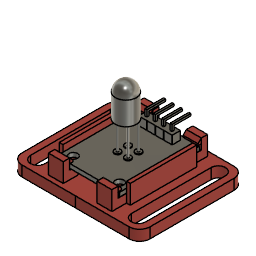
LED Holder (Autodesk Fusion 360 design; units mm, degrees)
Autodesk Fusion 360 part; units mm, degrees
note: some values were not read from the file. Chosen so that the rebuilt part matches the saved one: which bodies a step acts on; which face or edge a step refers to. Set by a fixed rule: which sketch regions a step uses.
sketch "Sketch1" plane through (0, 0, 0) normal (0, 0, 1) x (1, 0, 0)
  line L0 (0, 0) -> (15, 0)
  line L1 (15, 0) -> (15, 19)
  line L2 (15, 19) -> (0, 19)
  line L3 (0, 19) -> (0, 0)
  line L4 (0, 0) -> (2, 0) construction
  line L5 (2, 0) -> (2, 2) construction
  line L6 (2, 2) -> (0, 2) construction
  line L7 (0, 2) -> (0, 0) construction
  circle A0 centre (2, 2) radius 1
  circle A1 centre (13, 2) radius 1
  dimension "d1" = 15
  dimension "d2" = 19
  constraint horizontal L0
  constraint vertical L1
  constraint horizontal L2
  constraint vertical L3
  constraint coincident L0.start L3.end
  constraint horizontal L4
  constraint vertical L5
  constraint horizontal L6
  constraint vertical L7
  constraint coincident L5.end L6.start
  measures "d1" distance of L0.start L0.end
  measures "d2" distance of L0.start L2.end
extrude "Extrude1" add sketch "Sketch1" along normal blind 1 makes body 1
sketch "Sketch2" plane through (0, 0, 1) normal (0, 0, 1) x (-1, 0, 0)
  circle A0 centre (-13, -2) radius 1
  circle A1 centre (-2, -2) radius 1
  line L0 (0, -19) -> (0, 0)
  line L1 (0, 0) -> (-15, 0)
  line L2 (-15, 0) -> (-15, -19)
  line L3 (-15, -19) -> (0, -19)
  line L4 (-7.5, -19) -> (-7.5, -18) construction
  line L5 (-7.5, -18) -> (-7.5, -17) construction
  line L6 (-11.5, -18) -> (-3.5, -18)
  line L7 (-3.5, -18) -> (-3.5, -16)
  line L8 (-3.5, -16) -> (-11.5, -16)
  line L9 (-11.5, -16) -> (-11.5, -18)
  line L10 (-11.5, -18) -> (-3.5, -16) construction
  line L11 (-3.5, -18) -> (-11.5, -16) construction
  circle A2 centre (-3.5, -18) radius 0.05
  circle A3 centre (-5.5, -18) radius 0.05
  circle A4 centre (-7.5, -18) radius 0.05
  circle A5 centre (-9.5, -18) radius 0.05
  circle A6 centre (-11.5, -18) radius 0.05
  circle A7 centre (-3.5, -16) radius 0.05
  circle A8 centre (-5.5, -16) radius 0.05
  circle A9 centre (-7.5, -16) radius 0.05
  circle A10 centre (-9.5, -16) radius 0.05
  circle A11 centre (-11.5, -16) radius 0.05
  point P0 (-7.5, -17)
  dimension "d5" = 8
  dimension "d6" = 2
  dimension "d7" = 0.1
  dimension "d10" = -2
  dimension "d11" = 2
  constraint midpoint L3 L4.start
  constraint perpendicular L3 L4
  constraint parallel L4 L5
  constraint horizontal L6
  constraint perpendicular L6 L7
  constraint parallel L6 L8
  constraint parallel L7 L9
  constraint coincident L10 P0
  constraint coincident L11 P0
  constraint coincident P0 L5.end
  constraint coincident L6.end L7.start
  measures "d5" distance of L7.end L8.end
  measures "d6" distance of L6.end L7.end
  measures "d7" diameter of A2
extrude "Extrude2" add sketch "Sketch2" along normal blind 2 contours L6 L7 L8 L9 A2 A3 A4 A5 A6 A7 A8 A9 A10 A11 bodies 1
sketch "Sketch3" plane through (0, 0, 1) normal (0, 0, 1) x (-1, 0, 0)
  arc A0 (-7.55, -16) -> (-7.45, -16) centre (-7.5, -16) ccw
  line L0 (-7.45, -16) -> (-5.55, -16)
  arc A1 (-5.55, -16) -> (-5.45, -16) centre (-5.5, -16) ccw
  line L1 (-5.45, -16) -> (-3.55, -16)
  arc A2 (-3.55, -16) -> (-3.5, -16.05) centre (-3.5, -16) ccw
  line L2 (-3.5, -16.05) -> (-3.5, -17.95)
  arc A3 (-3.5, -17.95) -> (-3.55, -18) centre (-3.5, -18) ccw
  line L3 (-3.55, -18) -> (-5.45, -18)
  arc A4 (-5.45, -18) -> (-5.55, -18) centre (-5.5, -18) ccw
  line L4 (-5.55, -18) -> (-7.45, -18)
  arc A5 (-7.45, -18) -> (-7.55, -18) centre (-7.5, -18) ccw
  line L5 (-7.55, -18) -> (-9.45, -18)
  arc A6 (-9.45, -18) -> (-9.55, -18) centre (-9.5, -18) ccw
  line L6 (-9.55, -18) -> (-11.45, -18)
  arc A7 (-11.45, -18) -> (-11.5, -17.95) centre (-11.5, -18) ccw
  line L7 (-11.5, -17.95) -> (-11.5, -16.05)
  arc A8 (-11.5, -16.05) -> (-11.45, -16) centre (-11.5, -16) ccw
  line L8 (-11.45, -16) -> (-9.55, -16)
  arc A9 (-9.55, -16) -> (-9.45, -16) centre (-9.5, -16) ccw
  line L9 (-9.45, -16) -> (-7.55, -16)
  circle A10 centre (-13, -2) radius 1
  circle A11 centre (-2, -2) radius 1
  line L10 (0, -19) -> (0, 0)
  line L11 (0, 0) -> (-15, 0)
  line L12 (-15, 0) -> (-15, -19)
  line L13 (-15, -19) -> (0, -19)
  line L14 (-7.5, -19) -> (-7.5, -9) construction
  circle A12 centre (-7.5, -9) radius 2.5
  dimension "d14" = 10
  dimension "d15" = 5
  constraint midpoint L13 L14.start
  constraint perpendicular L13 L14
  constraint coincident L14.end A12.centre
  measures "d14" distance of L14.start L14.end
  measures "d15" diameter of A12
extrude "Extrude3" add sketch "Sketch3" along normal blind 15 contours A12 bodies 1
extrude "Extrude4" cut sketch "Sketch3" along normal blind 7 contours A12 bodies 1 makes body 2 at (5.8333, 13.622, 0)
fillet "Fillet1" radius 2.5 1 edges at (9.8308, 9.904, 16) on bodies 1
sketch "Sketch4" plane through (0, 0, 1) normal (0, 0, 1) x (-1, 0, 0)
  circle A0 centre (-6.5, -10.5) radius 0.75
  circle A1 centre (-6.5, -8) radius 0.75
  circle A2 centre (-9, -10.5) radius 0.75
  circle A3 centre (-9, -8) radius 0.75
  circle A4 centre (-6.5, -10.5) radius 0.25
  circle A5 centre (-6.5, -8) radius 0.25
  circle A6 centre (-9, -8) radius 0.25
  circle A7 centre (-9, -10.5) radius 0.25
  dimension "d22" = 1.5
  dimension "d23" = 1.5
  dimension "d24" = 1.5
  dimension "d25" = 1.5
  dimension "d26" = 0.5
  dimension "d27" = 0.5
  dimension "d28" = 0.5
  dimension "d29" = 0.5
  constraint concentric A0 A4
  constraint concentric A1 A5
  constraint concentric A3 A6
  constraint concentric A2 A7
  measures "d22" diameter of A0
  measures "d23" diameter of A1
  measures "d24" diameter of A2
  measures "d25" diameter of A3
  measures "d26" diameter of A4
  measures "d27" diameter of A5
  measures "d28" diameter of A6
  measures "d29" diameter of A7
extrude "Extrude5" add sketch "Sketch4" along normal blind 7 contours A4 | A5 | A6 | A7 bodies 1 2
extrude "Extrude7" add sketch "Sketch4" against normal blind 2 contours A4 | A5 | A6 | A7 bodies 1
extrude "Extrude8" add sketch "Sketch4" along normal blind 0.2 bodies 1
sketch "Sketch5" plane through (0, 0, 3) normal (0, 0, 1) x (-1, 0, 0)
  line L0 (-7.55, -16) -> (-9.45, -16)
  arc A0 (-9.55, -16) -> (-9.45, -16) centre (-9.5, -16) ccw
  line L1 (-9.55, -16) -> (-11.45, -16)
  arc A1 (-11.5, -16.05) -> (-11.45, -16) centre (-11.5, -16) ccw
  line L2 (-11.5, -16.05) -> (-11.5, -17.95)
  arc A2 (-11.45, -18) -> (-11.5, -17.95) centre (-11.5, -18) ccw
  line L3 (-11.45, -18) -> (-9.55, -18)
  arc A3 (-9.45, -18) -> (-9.55, -18) centre (-9.5, -18) ccw
  line L4 (-9.45, -18) -> (-7.55, -18)
  arc A4 (-7.45, -18) -> (-7.55, -18) centre (-7.5, -18) ccw
  line L5 (-7.45, -18) -> (-5.55, -18)
  arc A5 (-5.45, -18) -> (-5.55, -18) centre (-5.5, -18) ccw
  line L6 (-5.45, -18) -> (-3.55, -18)
  arc A6 (-3.5, -17.95) -> (-3.55, -18) centre (-3.5, -18) ccw
  line L7 (-3.5, -17.95) -> (-3.5, -16.05)
  arc A7 (-3.55, -16) -> (-3.5, -16.05) centre (-3.5, -16) ccw
  line L8 (-3.55, -16) -> (-5.45, -16)
  arc A8 (-5.55, -16) -> (-5.45, -16) centre (-5.5, -16) ccw
  line L9 (-5.55, -16) -> (-7.45, -16)
  arc A9 (-7.55, -16) -> (-7.45, -16) centre (-7.5, -16) ccw
  line L10 (-10.25, -16.75) -> (-10.75, -16.75)
  line L11 (-10.75, -16.75) -> (-10.75, -17.25)
  line L12 (-10.75, -17.25) -> (-10.25, -17.25)
  line L13 (-10.25, -17.25) -> (-10.25, -16.75)
  line L14 (-10.25, -16.75) -> (-10.75, -17.25) construction
  line L15 (-10.75, -16.75) -> (-10.25, -17.25) construction
  line L16 (-8.25, -17.25) -> (-8.25, -16.75)
  line L17 (-8.25, -16.75) -> (-8.75, -16.75)
  line L18 (-8.75, -16.75) -> (-8.75, -17.25)
  line L19 (-8.75, -17.25) -> (-8.25, -17.25)
  line L20 (-6.25, -17.25) -> (-6.25, -16.75)
  line L21 (-6.25, -16.75) -> (-6.75, -16.75)
  line L22 (-6.75, -16.75) -> (-6.75, -17.25)
  line L23 (-6.75, -17.25) -> (-6.25, -17.25)
  line L24 (-4.25, -17.25) -> (-4.25, -16.75)
  line L25 (-4.25, -16.75) -> (-4.75, -16.75)
  line L26 (-4.75, -16.75) -> (-4.75, -17.25)
  line L27 (-4.75, -17.25) -> (-4.25, -17.25)
  point P0 (-10.5, -17)
  dimension "d38" = 0.5
  dimension "d39" = 0.5
  dimension "d42" = 2
  dimension "d43" = 0
  constraint horizontal L10
  constraint perpendicular L10 L11
  constraint parallel L10 L12
  constraint parallel L11 L13
  constraint coincident L14 P0
  constraint coincident L15 P0
  measures "d38" distance of L11.end L12.end
  measures "d39" distance of L10.end L11.end
extrude "Extrude9" add sketch "Sketch5" along normal blind 1.5 contours L10 L11 L12 L13 | L16 L17 L18 L19 | L20 L21 L22 L23 | L24 L25 L26 L27 bodies 1
sketch "Sketch6" plane through (0, 17.25, 0) normal (0, 1, 0) x (-1, 0, 0)
  line L0 (-10.75, 3) -> (-10.25, 3)
  line L1 (-10.25, 3) -> (-10.25, 4.5)
  line L2 (-10.25, 4.5) -> (-10.75, 4.5)
  line L3 (-10.75, 4.5) -> (-10.75, 3)
  line L4 (-10.75, 4.5) -> (-10.25, 4.5)
  line L5 (-10.25, 4.5) -> (-10.25, 4)
  line L6 (-10.25, 4) -> (-10.75, 4)
  line L7 (-10.75, 4) -> (-10.75, 4.5)
  dimension "d46" = 0.5
  constraint horizontal L4
  constraint vertical L5
  constraint horizontal L6
  constraint vertical L7
  constraint coincident L2.end L3.start
  measures "d46" distance of L2.end L6.end
extrude "Extrude10" add sketch "Sketch6" along normal blind 4 contours L1 L2 L3 L4 L5 L6 L7 bodies 1
pattern_linear "R-Pattern1" count 4 spacing 2 along (-1, 0, 0) of "Extrude10"
sketch "Sketch7" plane through (0, 0, 0) normal (0, 0, -1) x (1, 0, 0)
  circle A0 centre (9, -10.5) radius 0.25
  circle A1 centre (9, -8) radius 0.25
  circle A2 centre (6.5, -10.5) radius 0.25
  circle A3 centre (6.5, -8) radius 0.25
  circle A4 centre (13, -2) radius 1
  circle A5 centre (2, -2) radius 1
  line L0 (0, 0) -> (0, -19)
  line L1 (0, -19) -> (15, -19)
  line L2 (15, -19) -> (15, 0)
  line L3 (15, 0) -> (0, 0)
  line L4 (7.5, 0) -> (-5.25, 0) construction
  line L5 (-5.25, 0) -> (7.5, 0)
  line L6 (7.5, -25) -> (-5.25, -25)
  line L7 (-7.75, -22.5) -> (-7.75, -2.5)
  line L8 (-7.75, -12.5) -> (-4.5, -12.5) construction
  line L9 (-2.8, -22) -> (-2.8, -3)
  arc A6 (-2.8, -3) -> (-6.2, -3) centre (-4.5, -3) ccw
  line L10 (-6.2, -3) -> (-6.2, -22)
  arc A7 (-6.2, -22) -> (-2.8, -22) centre (-4.5, -22) ccw
  line L11 (-4.5, -22) -> (-4.5, -3) construction
  line L12 (7.5, -25) -> (7.5, 0) construction
  arc A8 (-5.25, 0) -> (-7.75, -2.5) centre (-5.25, -2.5) ccw
  line L13 (0, 0) -> (7.5, 0) construction
  arc A9 (-7.75, -22.5) -> (-5.25, -25) centre (-5.25, -22.5) ccw
  line L14 (20.25, 0) -> (7.5, 0)
  arc A10 (22.75, -2.5) -> (20.25, 0) centre (20.25, -2.5) ccw
  line L15 (22.75, -22.5) -> (22.75, -2.5)
  arc A11 (20.25, -25) -> (22.75, -22.5) centre (20.25, -22.5) ccw
  line L16 (7.5, -25) -> (20.25, -25)
  arc A12 (17.8, -22) -> (21.2, -22) centre (19.5, -22) ccw
  line L17 (17.8, -22) -> (17.8, -3)
  line L18 (21.2, -3) -> (21.2, -22)
  arc A13 (21.2, -3) -> (17.8, -3) centre (19.5, -3) ccw
  line L19 (19.5, -22) -> (-4.5, -22) construction
  point P0 (-4.5, -12.5)
  dimension "d53" = 3.25
  dimension "d54" = 3.4
  dimension "d55" = 2.5
  dimension "d56" = 2.5
  dimension "d59" = 25
  dimension "d60" = 19
  dimension "d68" = 30.5
  dimension "d69" = 24
  constraint midpoint L3 L4.start
  constraint parallel L3 L4
  constraint perpendicular L2 L13
  constraint horizontal L5
  constraint horizontal L6
  constraint vertical L7
  constraint perpendicular L0 L8
  constraint tangent L9 A6
  constraint tangent A6 L10
  constraint parallel L9 L10
  constraint tangent L10 A7
  constraint tangent L9 A7
  constraint perpendicular L8 L11
  constraint coincident P0 L8.end
  constraint midpoint L11 P0
  constraint coincident L7 L8.start
  constraint tangent L5 A8
  constraint tangent L7 A8
  constraint coincident L0 L3.end
  constraint tangent L6 A9
  constraint tangent L7 A9
  constraint symmetric L4.start L12 L5.end
  constraint symmetric L9.start L12 A12.start
  constraint symmetric L9.end L12 L17.end
  constraint symmetric A6.end L12 L18.start
  constraint symmetric L10.end L12 A12.end
  constraint symmetric A6 L12 A13
  constraint symmetric A7 L12 A12
  constraint symmetric L6.start L12 L16.start
  constraint symmetric L12 L4.end L14.start
  constraint symmetric L12 L7.end A10.start
  constraint symmetric L12 A8 A10
  constraint symmetric L12 L6.end A11.start
  constraint symmetric L12 L7.start L15.start
  constraint symmetric L12 A9 A11
  constraint coincident A12.centre L19.start
  constraint coincident A7.centre L11.start
  measures "d53" distance of L8.start P0
  measures "d54" diameter of A6
  measures "d55" radius of A8
  measures "d56" radius of A9
  measures "d59" distance of L5 L6
  measures "d60" distance of A7.centre A6.centre
  measures "d68" distance of L7 L15
  measures "d69" distance of A12.centre A7.centre
extrude "Extrude11" add sketch "Sketch7" along normal blind 2.5 separate body contours A0 | A1 | A2 | A3 | A4 | A5 | L0 L1 L2 L3 L5 L14 | L0 L1 L2 L5 L6 L7 A8 A9 L14 A10 L15 A11 L16 makes body 3
move_body "Move1" bodies 1 to x (1, 0, 0) y (0, 1, 0) z (0, 0, 1) at (0, 3, 2)
sketch "Sketch8" plane through (0, 0, 0) normal (0, 0, 1) x (-1, 0, 0)
  arc A0 (2.8, -22) -> (6.2, -22) centre (4.5, -22) ccw
  line L0 (2.8, -22) -> (2.8, -3)
  arc A1 (6.2, -3) -> (2.8, -3) centre (4.5, -3) ccw
  line L1 (6.2, -3) -> (6.2, -22)
  arc A2 (-21.2, -22) -> (-17.8, -22) centre (-19.5, -22) ccw
  line L2 (-21.2, -22) -> (-21.2, -3)
  arc A3 (-17.8, -3) -> (-21.2, -3) centre (-19.5, -3) ccw
  line L3 (-17.8, -3) -> (-17.8, -22)
  arc A4 (5.25, -25) -> (7.75, -22.5) centre (5.25, -22.5) ccw
  line L4 (7.75, -22.5) -> (7.75, -2.5)
  arc A5 (7.75, -2.5) -> (5.25, 0) centre (5.25, -2.5) ccw
  line L5 (5.25, 0) -> (-7.5, 0)
  line L6 (-7.5, 0) -> (-20.25, 0)
  arc A6 (-20.25, 0) -> (-22.75, -2.5) centre (-20.25, -2.5) ccw
  line L7 (-22.75, -2.5) -> (-22.75, -22.5)
  arc A7 (-22.75, -22.5) -> (-20.25, -25) centre (-20.25, -22.5) ccw
  line L8 (-20.25, -25) -> (-7.5, -25)
  line L9 (-7.5, -25) -> (5.25, -25)
  line L10 (0.05, -20.4) -> (-3.5, -20.4)
  line L11 (-3.5, -20.4) -> (-3.5, -23.9)
  line L12 (-3.5, -23.9) -> (0.05, -23.9)
  line L13 (0.05, -23.9) -> (0.05, -20.4)
  line L14 (0.05, -23.9) -> (-3.5, -23.9)
  line L15 (-3.5, -23.9) -> (-3.5, -22.4)
  line L16 (-3.5, -22.4) -> (0.05, -22.4)
  line L17 (0.05, -22.4) -> (0.05, -23.9)
  line L18 (-7.5, -25) -> (-7.5, 0) construction
  line L19 (7.75, -12.5) -> (-22.75, -12.5) construction
  line L20 (-15.05, -20.4) -> (-11.5, -20.4)
  line L21 (-11.5, -20.4) -> (-11.5, -23.9)
  line L22 (-15.05, -23.9) -> (-15.05, -20.4)
  line L23 (-11.5, -23.9) -> (-15.05, -23.9)
  line L24 (-15.05, -23.9) -> (-11.5, -23.9)
  line L25 (-11.5, -23.9) -> (-11.5, -22.4)
  line L26 (-15.05, -22.4) -> (-15.05, -23.9)
  line L27 (-11.5, -22.4) -> (-15.05, -22.4)
  line L28 (0.05, -4.6) -> (-3.5, -4.6)
  line L29 (-3.5, -4.6) -> (-3.5, -1.1)
  line L30 (0.05, -1.1) -> (0.05, -4.6)
  line L31 (-3.5, -1.1) -> (0.05, -1.1)
  line L32 (0.05, -1.1) -> (-3.5, -1.1)
  line L33 (-3.5, -1.1) -> (-3.5, -2.6)
  line L34 (0.05, -2.6) -> (0.05, -1.1)
  line L35 (-3.5, -2.6) -> (0.05, -2.6)
  line L36 (-11.5, -1.1) -> (-11.5, -2.6)
  line L37 (-11.5, -2.6) -> (-15.05, -2.6)
  line L38 (-15.05, -2.6) -> (-15.05, -1.1)
  line L39 (-15.05, -1.1) -> (-11.5, -1.1)
  line L40 (-15.05, -1.1) -> (-15.05, -4.6)
  line L41 (-11.5, -4.6) -> (-11.5, -1.1)
  line L42 (-11.5, -1.1) -> (-15.05, -1.1)
  line L43 (-15.05, -4.6) -> (-11.5, -4.6)
  line L44 (0.05, -20.4) -> (0.95, -20.4)
  line L45 (0.95, -20.4) -> (0.95, -4.6)
  line L46 (0.95, -4.6) -> (0.05, -4.6)
  line L47 (0.05, -4.6) -> (0.05, -20.4)
  line L48 (0.05, -20.4) -> (0.95, -4.6) construction
  line L49 (0.95, -20.4) -> (0.05, -4.6) construction
  line L50 (-15.05, -20.4) -> (-15.95, -20.4)
  line L51 (-15.95, -20.4) -> (-15.95, -4.6)
  line L52 (-15.95, -4.6) -> (-15.05, -4.6)
  line L53 (-15.05, -4.6) -> (-15.05, -20.4)
  point P0 (0.5, -12.5)
  dimension "d70" = 0.9
  constraint horizontal L10
  constraint vertical L11
  constraint horizontal L12
  constraint vertical L13
  constraint horizontal L14
  constraint vertical L15
  constraint horizontal L16
  constraint vertical L17
  constraint coincident L8.end L9.start
  constraint coincident L5.end L6.start
  constraint midpoint L4 L19.start
  constraint midpoint L7 L19.end
  constraint symmetric L10.start L18 L20.start
  constraint symmetric L10.end L18 L20.end
  constraint symmetric L11.end L18 L21.end
  constraint symmetric L12.end L18 L22.start
  constraint symmetric L15.end L18 L25.end
  constraint symmetric L16.end L18 L26.start
  constraint symmetric L10.start L19 L28.start
  constraint symmetric L10.end L19 L28.end
  constraint symmetric L11.end L19 L29.end
  constraint symmetric L12.end L19 L30.start
  constraint symmetric L15.end L19 L33.end
  constraint symmetric L16.end L19 L34.start
  constraint symmetric L19 L20.start L40.end
  constraint symmetric L19 L20.end L41.start
  constraint symmetric L19 L21.end L36.start
  constraint symmetric L19 L22.start L38.end
  constraint symmetric L19 L25.end L36.end
  constraint symmetric L19 L26.start L37.end
  constraint horizontal L44
  constraint perpendicular L44 L45
  constraint parallel L44 L46
  constraint parallel L45 L47
  constraint coincident L48 P0
  constraint coincident L49 P0
  constraint coincident L19 P0
  constraint symmetric L18 L44.end L50.end
  constraint symmetric L18 L45.end L51.end
  constraint symmetric L18 L28.start L40.end
  measures "d70" distance of L45 L47
extrude "Extrude12" add sketch "Sketch8" along normal blind 2 contours L10 L11 L13 L16 | L28 L29 L30 L35 | L20 L21 L22 L27 | L37 L40 L41 L43 bodies 3
extrude "Extrude13" add sketch "Sketch8" along normal blind 4.5 contours L44 L45 L46 L47 | L11 L12 L13 L14 L15 L16 L17 | L29 L30 L31 L32 L33 L34 L35 | L50 L51 L52 L53 | L21 L22 L23 L24 L25 L26 L27 | L36 L37 L38 L39 L40 L41 L42 bodies 3
sketch "Sketch9" plane through (0, 0, 4.5) normal (0, 0, 1) x (-1, 0, 0)
  line L0 (-11.5, -22.4) -> (-15.05, -22.4)
  line L1 (-15.05, -22.4) -> (-15.05, -23.9)
  line L2 (-15.05, -23.9) -> (-11.5, -23.9)
  line L3 (-11.5, -23.9) -> (-11.5, -22.4)
  line L4 (-15.05, -22.4) -> (-11.4939, -22.4)
  line L5 (-11.4939, -22.4) -> (-11.4939, -21.5995)
  line L6 (-11.4939, -21.5995) -> (-15.05, -21.5995)
  line L7 (-15.05, -21.5995) -> (-15.05, -22.4)
  line L8 (-7.5, -25) -> (-7.5, 0) construction
  line L9 (0.05, -22.4) -> (-3.5061, -22.4)
  line L10 (-3.5061, -22.4) -> (-3.5061, -21.5995)
  line L11 (0.05, -21.5995) -> (0.05, -22.4)
  line L12 (-3.5061, -21.5995) -> (0.05, -21.5995)
  line L13 (-7.5, -12.5) -> (2.7337, -12.5) construction
  line L14 (0.05, -2.6) -> (-3.5061, -2.6)
  line L15 (-3.5061, -2.6) -> (-3.5061, -3.4005)
  line L16 (0.05, -3.4005) -> (0.05, -2.6)
  line L17 (-3.5061, -3.4005) -> (0.05, -3.4005)
  line L18 (-15.05, -2.6) -> (-11.4939, -2.6)
  line L19 (-11.4939, -2.6) -> (-11.4939, -3.4005)
  line L20 (-15.05, -3.4005) -> (-15.05, -2.6)
  line L21 (-11.4939, -3.4005) -> (-15.05, -3.4005)
  constraint horizontal L4
  constraint vertical L5
  constraint horizontal L6
  constraint vertical L7
  constraint coincident L0.end L1.start
  constraint perpendicular L2 L8
  constraint symmetric L0.end L8 L9.start
  constraint symmetric L4.end L8 L9.end
  constraint symmetric L5.end L8 L10.end
  constraint symmetric L6.end L8 L11.start
  constraint midpoint L8 L13.start
  constraint perpendicular L8 L13
  constraint symmetric L0.end L13 L18.start
  constraint symmetric L4.end L13 L18.end
  constraint symmetric L5.end L13 L19.end
  constraint symmetric L6.end L13 L20.start
  constraint symmetric L9.start L13 L14.start
  constraint symmetric L9.end L13 L14.end
  constraint symmetric L10.end L13 L15.end
  constraint symmetric L11.start L13 L16.start
extrude "Extrude14" add sketch "Sketch9" against normal blind 1.2 contours L0 L4 L5 L6 L7 | L9 L10 L11 L12 | L14 L15 L16 L17 | L18 L19 L20 L21 bodies 3
chamfer "Chamfer1" distance 0.8 angle 45 4 edges at (13.272, 21.5995, 4.5) (1.728, 21.5995, 4.5) (13.272, 3.4005, 4.5) (1.728, 3.4005, 4.5) on bodies 3
equation "d5 = ( 2 * 4 ) * 1 mm"
equation "d53 = ( 6.5 / 2 ) * 1 mm"
named bodies: "LED Holder"
